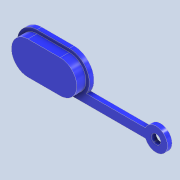
# Autodesk Inventor part: tappino tpu
Saved by Autodesk Inventor 2022 (Build 260153000, 153)
## iProperties
Created: 2025-08-17
Part Number: tappino tpu
Material: Thermoplastic Resin
Document SubType Name: Modeling
Designer: sacchie
Density: 1.28 g/cm^3
Appearance: Smooth - Black
Author: sacchie
Autodesk Inventor part; units mm, degrees
ref_plane "YZ Plane" through (0, 0, 0) normal (1, 0, 0) x (0, 1, 0)
ref_plane "XZ Plane" through (0, 0, 0) normal (0, 1, 0) x (-1, 0, 0)
ref_plane "XY Plane" through (0, 0, 0) normal (0, 0, 1) x (1, 0, 0)
sketch "Sketch1" plane through (0, 0, 0) normal (0, 0, 1) x (1, 0, 0)
  line L0 (0, 0) -> (-7, 0) construction
  line L1 (0, 4.35) -> (-7, 4.35)
  line L2 (-7, -4.35) -> (0, -4.35)
  arc A0 (0, -4.35) -> (0, 4.35) centre (0, 0) ccw
  arc A1 (-7, 4.35) -> (-7, -4.35) centre (-7, 0) ccw
  line L3 (-7, 3.6) -> (0, 3.6)
  arc A2 (0, -3.6) -> (0, 3.6) centre (0, 0) ccw
  line L4 (0, -3.6) -> (-7, -3.6)
  arc A3 (-7, 3.6) -> (-7, -3.6) centre (-7, 0) ccw
  line L5 (0, -4.35) -> (19.2, -4.35)
  line L6 (20, -3.55) -> (20, -3.15)
  line L7 (19.2, -2.35) -> (3.6606, -2.35)
  circle A4 centre (18.8, -3.35) radius 1
  arc A5 (20, -3.15) -> (19.2, -2.35) centre (19.2, -3.15) ccw
  arc A6 (19.2, -4.35) -> (20, -3.55) centre (19.2, -3.55) ccw
  arc A7 (16.5087, -4.35) -> (16.5087, -2.35) centre (18.8, -3.35) ccw
  line L8 (18.8, -3.35) -> (5.3494, -3.35) construction
  point P0 (-3.5, 0)
  point P1 (20, -4.35)
  point P2 (20, -2.35)
  dimension "d0" = 7
  dimension "d1" = 8.7
  dimension "d5" = 3.6
  dimension "d6" = 2
  dimension "d7" = 2
  dimension "d8" = 20
  dimension "d9" = 1.2
  dimension "d10" = 0.8
  dimension "d13" = 5
  dimension "d14" = 1
  constraints: 20 end point, 15 point on circle, 8 centre point, 8 tangent, 6 point on line, 3 parallel, 2 horizontal, 2 perpendicular, 1 coincident, 1 equal radius, 1 midpoint, 3 other
  measures "d0" distance of L0.start L0.end
  measures "d1" diameter of A1
  measures "d5" radius of A2
  measures "d6" distance of point (20, -4.35) point (20, -2.35)
  measures "d7" diameter of A4
  measures "d8" distance from line of L0.start L6
  measures "d9" distance from line of L6 A4.centre
  measures "d10" radius of A5
  measures "d13" diameter of A7
  measures "d14" distance between parallel lines of L7 L8
extrude "Extrusion1" add sketch "Sketch1" along normal blind 1 contours A0 L2 A1 L1 | L7 A4 L5 A0 | A7 L5 A6 L6 A5 L7 | L7 A5 L6 A6 L5 A4 | L3 A2 L4 A3
extrude "Extrusion2" add sketch "Sketch1" along normal blind 2 from surface at 1 contours L3 A2 L4 A3
body "Solid1"
